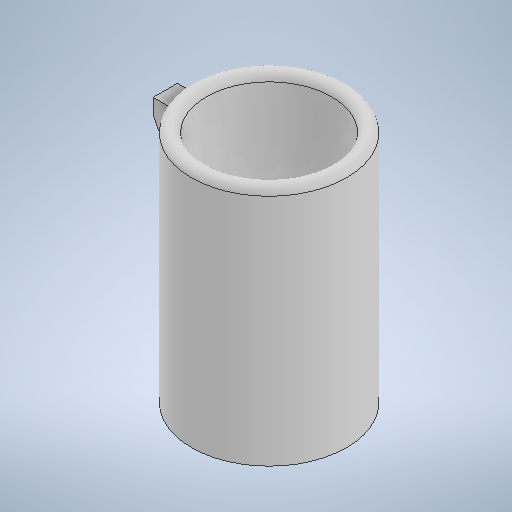
# Autodesk Inventor part: cap
Saved by Autodesk Inventor 2025 (Build 290162000, 162)
## iProperties
Created: 2025-03-25
Part Number: cap
Material: Generic
Document SubType Name: Modeling
Designer: ethan
Density: 1 g/cm^3
Appearance: Default
Author: ethan
Autodesk Inventor part; units mm, degrees
ref_plane "YZ Plane" through (0, 0, 0) normal (1, 0, 0) x (0, 1, 0)
ref_plane "XZ Plane" through (0, 0, 0) normal (0, 1, 0) x (-1, 0, 0)
ref_plane "XY Plane" through (0, 0, 0) normal (0, 0, 1) x (1, 0, 0)
sketch "Sketch1" plane through (0, 0, 0) normal (0, 1, 0) x (-1, 0, 0)
  circle A0 centre (0, 0) radius 16.75 construction
  circle A1 centre (0, 0) radius 16.75
  circle A2 centre (0, 0) radius 20.75
  dimension "d0" = 33.5
  dimension "d1" = 4
  constraints: 3 centre point, 2 coincident, 1 concentric
  measures "d0" diameter of A0
  measures "d1" radial gap between concentric circles of A0 A2
extrude "Extrusion1" add sketch "Sketch1" along normal blind 55
ref_plane "Work Plane1" through (0, 27.5, 0) normal (0, 1, 0) x (1, 0, 0)
sketch "Sketch2" plane through (0, 27.5, 0) normal (0, 1, 0) x (1, 0, 0)
  circle A0 centre (0, 0) radius 16.75 projected
  circle A1 centre (0, 0) radius 16.15
  dimension "d4" = 0.6
  constraints: 1 centre point
  measures "d4" radial gap between concentric circles of A0 A1
extrude "Extrusion2" add sketch "Sketch2" along normal mid plane 1
sketch "Sketch3" plane through (0, 0, 0) normal (0, -1, 0) x (1, 0, 0)
  circle A0 centre (0, 0) radius 20.75 projected
  circle A1 centre (0, 0) radius 16.75 projected
extrude "Extrusion3" add sketch "Sketch3" along normal blind 3.5
sketch "Sketch4" plane through (0, 55, 0) normal (0, 1, 0) x (1, 0, 0)
  circle A0 centre (0, 0) radius 20.75 construction
  circle A1 centre (0, 0) radius 16.75 construction
  line L0 (-13.75, -3.25) -> (-13.75, 3.25) construction
  line L1 (-13.75, 3.25) -> (-27.75, 3.25) construction
  line L2 (-27.75, 3.25) -> (-27.75, -3.25) construction
  line L3 (-27.75, -3.25) -> (-13.75, -3.25) construction
  line L4 (-13.75, -3.25) -> (-27.75, 3.25) construction
  line L5 (-13.75, 3.25) -> (-27.75, -3.25) construction
  line L6 (-20.4939, -3.25) -> (-27.75, -3.25)
  line L7 (-27.75, -3.25) -> (-27.75, 3.25)
  line L8 (-27.75, 3.25) -> (-20.4939, 3.25)
  arc A2 (-20.4939, 3.25) -> (-20.4939, -3.25) centre (0, 0) ccw
  point P0 (-20.75, 0)
  dimension "d10" = 6.5
  dimension "d11" = 14
  constraints: 18 end point, 6 point on circle, 3 equal length, 2 midpoint, 2 perpendicular, 2 point on line, 1 centre point, 1 vertical
  measures "d10" distance of L0.start L0.end
  measures "d11" distance of L1.end L0.end
extrude "Extrusion4" add sketch "Sketch4" against normal blind 12
chamfer "Chamfer1" distance 4 distance2 8 1 edges at (-27.75, 43, 0) measured on face at (-27.25, 43, 0)
sketch "Sketch5" plane through (0, 55, 0) normal (0, 1, 0) x (1, 0, 0)
  arc A0 (-20.4939, -3.25) -> (-20.4939, 3.25) centre (0, 0) ccw construction
  line L0 (-20.4939, 3.25) -> (-27.75, 3.25) construction
  line L1 (-27.75, 3.25) -> (-27.75, -3.25) construction
  line L2 (-27.75, -3.25) -> (-20.4939, -3.25) construction
  circle A1 centre (0, 0) radius 16.75 construction
  circle A2 centre (0, 0) radius 20.75
  circle A3 centre (0, 0) radius 16.75
  constraints: 2 coincident, 1 centre point, 3 other
extrude "Extrusion5" add sketch "Sketch5" along normal blind 6
fillet "Fillet2" radius 2 2 edges at (-20.75, 61, 0) (-16.75, 61, 0)
body "Solid1"
